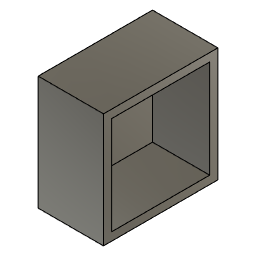
3D-модель манипулятора (Autodesk Fusion 360 archive; units mm, degrees)
design "Контейнер"
Autodesk Fusion 360 part; units mm, degrees
sketch "Sketch1" plane through (0, 0, 0) normal (1, 0, 0) x (0, 1, 0)
  line L0 (-35, 35) -> (35, 35)
  line L1 (35, 35) -> (35, -35)
  line L2 (35, -35) -> (-35, -35)
  line L3 (-35, -35) -> (-35, 35)
  line L4 (-35, 35) -> (35, -35) construction
  line L5 (35, 35) -> (-35, -35) construction
  dimension "d1" = 70
  dimension "d2" = 70
  constraint horizontal L0
  constraint perpendicular L0 L1
  constraint parallel L0 L2
  constraint parallel L1 L3
  constraint coincident L4 origin
  constraint coincident L5 origin
  measures "d1" distance of L0.end L1.end
  measures "d2" distance of L1.end L2.end
extrude "Extrude1" add sketch "Sketch1" along normal blind 40
sketch "Sketch2" plane through (40, 0, 0) normal (1, 0, 0) x (0, 1, 0)
  line L0 (-35, -35) -> (35, -35)
  line L1 (35, -35) -> (35, 35)
  line L2 (35, 35) -> (-35, 35)
  line L3 (-35, 35) -> (-35, -35)
  line L4 (-30, 30) -> (30, 30)
  line L5 (30, 30) -> (30, -30)
  line L6 (30, -30) -> (-30, -30)
  line L7 (-30, -30) -> (-30, 30)
  line L8 (-30, 30) -> (30, -30) construction
  line L9 (30, 30) -> (-30, -30) construction
  dimension "d5" = 5
  dimension "d6" = 5
  constraint horizontal L4
  constraint perpendicular L4 L5
  constraint parallel L4 L6
  constraint parallel L5 L7
  constraint coincident L8 origin
  constraint coincident L9 origin
  measures "d5" distance of L2 L4
  measures "d6" distance of L3 L7
extrude "Extrude2" cut sketch "Sketch2" against normal blind 35 contours L4 L5 L6 L7
